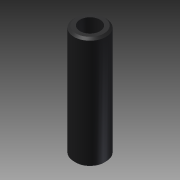
# Autodesk Inventor part: D-015
Saved by Autodesk Inventor 2015 (Build 190159000, 159)
## iProperties
Company: MARCHA TECHNOLOGY
Created: 2013-06-14
Part Number: D-015
Document SubType Name: Modeling
Designer: O.Martin
Density: 2.71 g/cm^3
Material: Aluminum-6061
Description: CASQUILLO SUPLEMENTO TRASMISION
Stock Number: 28448
Mass: 2.30793 g
Surface Area: 11.8943 cm^2
Volume: 0.851633 cm^3
Project: WITBOXprinter_V1.0
Appearance: Rubber - Black - Version 1.1
Author: O.Martin
Autodesk Inventor part; units mm, degrees
ref_plane "YZ Plane" through (0, 0, 0) normal (1, 0, 0) x (0, 1, 0)
ref_plane "XZ Plane" through (0, 0, 0) normal (0, 1, 0) x (-1, 0, 0)
ref_plane "XY Plane" through (0, 0, 0) normal (0, 0, 1) x (1, 0, 0)
sketch "Boceto1" plane through (0, 0, 0) normal (0, 0, 1) x (1, 0, 0)
  circle A0 centre (0, 0) radius 4
  circle A1 centre (0, 0) radius 2.5
  dimension "d0" = 5
  dimension "d1" = 8
  constraints: 2 centre point, 2 coincident
  measures "d0" diameter of A1
  measures "d1" diameter of A0
extrude "Extrusión1" add sketch "Boceto1" along normal blind 28
chamfer "Chaflán1" distance 0.5 angle 45 2 edges at (-4, 0, 28) (-4, 0, 0)
body "Solid1"
